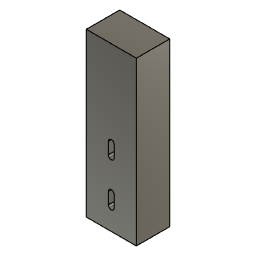
Hokey Seitenhalterung v3 (Autodesk Fusion 360 design; units mm, degrees)
Autodesk Fusion 360 part; units mm, degrees
sketch "Skizze1" plane through (0, 0, 0) normal (0, 0, 1) x (1, 0, 0)
  line L0 (30, 20) -> (-30, 20)
  line L1 (-30, 20) -> (-30, -20)
  line L2 (-30, -20) -> (30, -20)
  line L3 (30, -20) -> (30, 20)
  line L4 (30, 20) -> (-30, -20) construction
  line L5 (-30, 20) -> (30, -20) construction
  dimension "d2" = 60
  dimension "d3" = 40
  constraint perpendicular L0 L1
  constraint parallel L0 L2
  constraint parallel L1 L3
  constraint horizontal L0
  constraint coincident L4 origin
  constraint coincident L5 origin
  measures "d2" distance of L1.end L2.end
  measures "d3" distance of L0.end L1.end
extrude "Extrusion1" add sketch "Skizze1" along normal blind 195
sketch "Skizze3" plane through (0, -20, 0) normal (0, -1, 0) x (1, 0, 0)
  line L0 (-30, 0) -> (30, 0)
  line L1 (30, 0) -> (30, 195)
  line L2 (30, 195) -> (-30, 195)
  line L3 (-30, 195) -> (-30, 0)
  line L4 (-3.5, 40) -> (-3.5, 26)
  arc A0 (-3.5, 26) -> (3.5, 26) centre (0, 26) ccw
  line L5 (3.5, 26) -> (3.5, 40)
  arc A1 (3.5, 40) -> (-3.5, 40) centre (0, 40) ccw
  line L6 (0, 40) -> (0, 26) construction
  line L7 (-3.5, 92) -> (-3.5, 78)
  arc A2 (-3.5, 78) -> (3.5, 78) centre (0, 78) ccw
  line L8 (3.5, 78) -> (3.5, 92)
  arc A3 (3.5, 92) -> (-3.5, 92) centre (0, 92) ccw
  line L9 (0, 92) -> (0, 78) construction
  point P0 (0, 195)
  dimension "d6" = 14
  dimension "d7" = 7
  dimension "d8" = 14
  dimension "d9" = 7
  constraint tangent L4 A0
  constraint tangent A0 L5
  constraint parallel L4 L5
  constraint tangent L5 A1
  constraint tangent L4 A1
  constraint vertical L6
  constraint midpoint L2 P0
  constraint vertical A1.centre P0
  constraint tangent L7 A2
  constraint tangent A2 L8
  constraint parallel L7 L8
  constraint tangent L8 A3
  constraint tangent L7 A3
  constraint vertical L9
  constraint vertical P0 A3.centre
  measures "d6" distance of A1.centre A0.centre
  measures "d7" diameter of A0
  measures "d8" distance of A3.centre A2.centre
  measures "d9" diameter of A2
extrude "Extrusion2" cut sketch "Skizze3" against normal blind 40 contours L4 A0 L5 A1 | L7 A2 L8 A3
